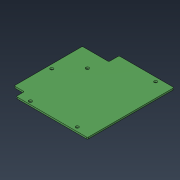
# Autodesk Inventor part: Mainboard
Saved by Autodesk Inventor 2022.1 (Build 261234020, 234B)
## iProperties
Part Number: Mainboard
Material: Phenolharz
Document SubType Name: Modeling
Designer: rYan
Mass: 14.1794 g
Surface Area: 134.436 cm^2
Volume: 10.275 cm^3
Density: 1.38 g/cm^3
Appearance: Glatt - waldgrün
Author: rYan
Autodesk Inventor part; units mm, degrees
ref_plane "YZ Plane" through (0, 0, 0) normal (1, 0, 0) x (0, 1, 0)
ref_plane "XZ Plane" through (0, 0, 0) normal (0, 1, 0) x (-1, 0, 0)
ref_plane "XY Plane" through (0, 0, 0) normal (0, 0, 1) x (1, 0, 0)
sketch "Skizze1" plane through (0, 0, 0) normal (0, 0, 1) x (1, 0, 0)
  line L0 (-10, -35) -> (70, -35)
  line L1 (70, -35) -> (70, 50)
  line L2 (70, 50) -> (-10, 50)
  line L3 (-10, 50) -> (-10, -35)
  line L4 (0, 67) -> (0, -52) projected
  line L5 (-26, 0) -> (86, 0) projected
  dimension "d0" = 80
  dimension "d1" = 85
  dimension "d4" = 35
  dimension "d5" = 10
  constraints: 8 end point, 2 parallel, 1 horizontal, 1 perpendicular
  measures "d0" distance of L2.end L1.end
  measures "d1" distance of L0.end L1.end
  measures "d4" distance between parallel lines of L5 L0
  measures "d5" distance between parallel lines of L3 L4
extrude "Extrusion1" add sketch "Skizze1" along normal blind 1.6
sketch "Skizze3" plane through (0, 0, 1.6) normal (0, 0, 1) x (1, 0, 0)
  line L0 (-10, -35) -> (70, -35) projected
  line L1 (70, -35) -> (70, 50) projected
  line L2 (70, 50) -> (-10, 50) projected
  line L3 (-10, 50) -> (-10, -35) projected
  line L4 (-10, -35) -> (0, -35)
  line L5 (0, -35) -> (0, -27)
  line L6 (0, -27) -> (-10, -27)
  line L7 (-10, -27) -> (-10, -35)
  line L8 (70, 50) -> (-10, 50) projected
  line L9 (-10, 50) -> (16, 50)
  line L10 (16, 50) -> (16, 40)
  line L11 (16, 40) -> (-10, 40)
  line L12 (-10, 40) -> (-10, 50)
  point P0 (0, 0)
  dimension "d19" = 10
  dimension "d20" = 8
  dimension "d23" = 26
  dimension "d24" = 10
  constraints: 16 end point, 4 parallel, 2 horizontal, 2 perpendicular
  measures "d19" distance of L5.end L6.end
  measures "d20" distance of L4.end L5.end
  measures "d23" distance of L10.end L11.end
  measures "d24" distance of L9.end L10.end
extrude "Extrusion2" cut sketch "Skizze3" against normal through all contours L3 L6 L5 L0 | L3 L2 L10 L11
sketch "Skizze2" plane through (0, 0, 1.6) normal (0, 0, 1) x (1, 0, 0)
  line L0 (-26, 0) -> (86, 0) projected
  line L1 (0, 67) -> (0, -52) projected
  point P0 (0, 0)
  point P1 (56, 46)
  point P2 (56, -31)
  point P3 (-6, 6)
  dimension "d13" = 56
  dimension "d14" = 46
  dimension "d15" = 6
  dimension "d17" = 31
  dimension "d18" = 56
  dimension "d35" = 6
  measures "d13" distance from line of point (56, 46) L1
  measures "d14" distance from line of point (56, 46) L0
  measures "d15" distance from line of point (-6, 6) L1
  measures "d17" distance from line of L0 point (56, -31)
  measures "d18" distance from line of L1 point (56, -31)
  measures "d35" distance from line of L0 point (-6, 6)
hole "Montage" at (56, 46, 1.6) at (56, -31, 1.6) at (-6, 6, 1.6) direction (0, 0, -1) diameter 3 end through all
sketch "Skizze4" plane through (0, 0, 1.6) normal (0, 0, 1) x (1, 0, 0)
  line L0 (0, 67) -> (0, -52) projected
  line L1 (-26, 0) -> (86, 0) projected
  line L2 (11, -32) -> (11, 24) construction
  point P0 (0, 0)
  dimension "d25" = 11
  dimension "d26" = 32
  dimension "d27" = 56
  constraints: 2 coincident, 2 end point, 1 vertical
  measures "d25" distance between parallel lines of L0 L2
  measures "d26" distance from line of point (11, -32) L1
  measures "d27" distance of L2.start L2.end
hole "Display" at (11, 24, 1.6) at (11, -32, 1.6) direction (0, 0, -1) diameter 3.2 end through all
fillet "Rundung1" radius 1 8 edges at (-10, -27, 0.8) (0, -27, 0.8) (0, -35, 0.8) (70, -35, 0.8) (70, 50, 0.8) (16, 50, 0.8) (16, 40, 0.8) (-10, 40, 0.8)
